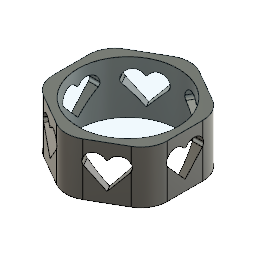
v3 v1 (Autodesk Fusion 360 design; units mm, degrees)
Autodesk Fusion 360 part; units mm, degrees
note: some values were not read from the file. Set by a fixed rule: which sketch regions a step uses.
sketch "Sketch1" plane through (0, 0, 0) normal (0, 1, 0) x (1, 0, 0)
  circle A0 centre (0, 0) radius 9.5
  circle A1 centre (0, 0) radius 12.5
  dimension "d1" = 19
  dimension "d2" = 25
  constraint coincident A0.centre A1.centre
  measures "d1" diameter of A0
  measures "d2" diameter of A1
extrude "Extrude1" add sketch "Sketch1" along normal blind 5 and the other way blind 5
sketch "Sketch2" plane through (0, 0, 0) normal (1, 0, 0) x (0, 0, -1)
  line L0 (3.2645, 0.6679) -> (0.0065, -3.0064)
  line L1 (0.0065, -3.0064) -> (-3.2632, 0.6658)
  arc A0 (3.5137, 1.4026) -> (0.2561, 2.1944) centre (1.7582, 1.2773) ccw
  arc A1 (-0.2561, 2.1944) -> (-3.5138, 1.4011) centre (-1.7582, 1.2773) ccw
  arc A2 (-3.5138, 1.4011) -> (-3.2632, 0.6658) centre (-2.5163, 1.3308) ccw
  arc A3 (3.2645, 0.6679) -> (3.5137, 1.4026) centre (2.5163, 1.3314) ccw
  arc A4 (-0.2561, 2.1944) -> (0.2561, 2.1944) centre (0, 2.3507) ccw
  dimension "d16" = 0.3
  constraint tangent A1 A2
  constraint tangent L1 A2
  constraint tangent A0 A3
  constraint tangent L0 A3
  constraint tangent A1 A4
  constraint tangent A0 A4
  measures "d16" radius of A4
extrude "Extrude2" cut sketch "Sketch2" along normal through all and the other way through all
pattern_circular "C-Pattern1" count 3 over 360 about axis through (0, 1.75, 0) along (0, 1, 0) of "Extrude2"
sketch "Sketch5" plane through (0, 5, 0) normal (0, 1, 0) x (-1, 0, 0)
  circle A0 centre (0, 0) radius 9.5
  circle A1 centre (0, 0) radius 12.5
  circle A2 centre (0.0007, 12.5) radius 1
  dimension "d20" = 2
  constraint coincident A1 A2.centre
  measures "d20" diameter of A2
extrude "Extrude3" add sketch "Sketch5" against normal up to surface (10 mm away) contours A1 A2 picked at (-0.0059, 12.8303)
fillet "Fillet1" radius 0.5 2 edges at (0.9985, 0, 12.4601) (-0.9999, 0, 12.4599)
pattern_circular "C-Pattern2" count 6 over 360 about axis through (0, 1.75, 0) along (0, 1, 0) of "Extrude3"
sketch "Sketch6" plane through (0, 5, 0) normal (0, 1, 0) x (-1, 0, 0)
  circle A0 centre (0, 0) radius 9.5
  arc A1 (-1.3839, 12.4232) -> (-10.2907, 7.0959) centre (0, 0) ccw
  arc A2 (-10.2907, 7.0959) -> (-11.29, 5.3653) centre (-10.825, 6.2506) ccw
  arc A3 (-11.29, 5.3653) -> (-11.2906, -5.364) centre (0, 0) ccw
  arc A4 (-11.2906, -5.364) -> (-10.2915, -7.0947) centre (-10.8257, -6.2494) ccw
  arc A5 (-10.2915, -7.0947) -> (-0.9999, -12.4599) centre (0, 0) ccw
  arc A6 (-0.9999, -12.4599) -> (0.9985, -12.4601) centre (-0.0007, -12.5) ccw
  arc A7 (0.9985, -12.4601) -> (10.2907, -7.0959) centre (0, 0) ccw
  arc A8 (10.2907, -7.0959) -> (11.29, -5.3653) centre (10.825, -6.2506) ccw
  arc A9 (11.29, -5.3653) -> (11.2906, 5.364) centre (0, 0) ccw
  arc A10 (11.2906, 5.364) -> (10.2915, 7.0947) centre (10.8257, 6.2494) ccw
  arc A11 (10.2915, 7.0947) -> (1.3853, 12.423) centre (0, 0) ccw
  arc A12 (0.9607, 12.7799) -> (1.3853, 12.423) centre (1.4407, 12.9199) ccw
  arc A13 (0.9607, 12.7799) -> (-0.9593, 12.7801) centre (0.0007, 12.5) ccw
  arc A14 (-1.3839, 12.4232) -> (-0.9593, 12.7801) centre (-1.4393, 12.9201) ccw
  line L0 (-2.5006, -11.0565) -> (-8.3258, -7.6929)
  line L1 (-10.8255, -3.3626) -> (-10.8251, 3.3639)
  line L2 (-8.3249, 7.6938) -> (-2.4994, 11.0568)
  line L3 (2.5006, 11.0565) -> (8.3258, 7.6929)
  line L4 (10.8255, 3.3626) -> (10.8251, -3.3639)
  line L5 (8.3249, -7.6938) -> (2.4994, -11.0568)
  arc A15 (-2.5006, -11.0565) -> (2.4994, -11.0568) centre (-0.0004, -6.7265) ccw
  arc A16 (-10.8255, -3.3626) -> (-8.3258, -7.6929) centre (-5.8255, -3.3629) ccw
  arc A17 (-8.3249, 7.6938) -> (-10.8251, 3.3639) centre (-5.8251, 3.3636) ccw
  arc A18 (2.5006, 11.0565) -> (-2.4994, 11.0568) centre (0.0004, 6.7265) ccw
  arc A19 (8.3249, -7.6938) -> (10.8251, -3.3639) centre (5.8251, -3.3636) ccw
  arc A20 (10.8255, 3.3626) -> (8.3258, 7.6929) centre (5.8255, 3.3629) ccw
  dimension "d27" = 5
  dimension "d28" = 5
  dimension "d29" = 5
  constraint tangent L5 A15
  constraint tangent L0 A15
  constraint tangent L0 A16
  constraint tangent L1 A16
  constraint equal A15 A16
  constraint tangent L1 A17
  constraint tangent L2 A17
  constraint equal A15 A17
  constraint tangent L2 A18
  constraint tangent L3 A18
  constraint equal A15 A18
  constraint tangent L5 A19
  constraint tangent L4 A19
  constraint tangent L4 A20
  constraint tangent L3 A20
  measures "d27" radius of A15
  measures "d28" radius of A19
  measures "d29" radius of A20
extrude "Extrude4" cut sketch "Sketch6" against normal blind 10 contours A1 A2 A3 A4 A5 A6 A7 A8 A9 A10 A11 A12 A13 A14
sketch "Sketch7" plane through (0, 5, 0) normal (0, 1, 0) x (-1, 0, 0)
  line L0 (2.4994, -11.0568) -> (8.3249, -7.6938)
  arc A0 (8.3249, -7.6938) -> (10.8251, -3.3639) centre (5.8251, -3.3636) ccw
  line L1 (10.8251, -3.3639) -> (10.8255, 3.3626)
  arc A1 (10.8255, 3.3626) -> (8.3258, 7.6929) centre (5.8255, 3.3629) ccw
  line L2 (8.3258, 7.6929) -> (2.5006, 11.0565)
  arc A2 (2.5006, 11.0565) -> (-2.4994, 11.0568) centre (0.0004, 6.7265) ccw
  line L3 (-2.4994, 11.0568) -> (-8.3249, 7.6938)
  arc A3 (-8.3249, 7.6938) -> (-10.8251, 3.3639) centre (-5.8251, 3.3636) ccw
  line L4 (-10.8251, 3.3639) -> (-10.8255, -3.3626)
  arc A4 (-10.8255, -3.3626) -> (-8.3258, -7.6929) centre (-5.8255, -3.3629) ccw
  line L5 (-8.3258, -7.6929) -> (-2.5006, -11.0565)
  arc A5 (-2.5006, -11.0565) -> (2.4994, -11.0568) centre (-0.0004, -6.7265) ccw
  circle A6 centre (0, 0) radius 9.5
